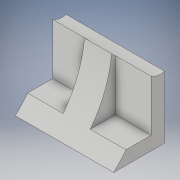
# Autodesk Inventor part: BottomRamp
Saved by Autodesk Inventor 2019 (Build 230136000, 136)
## iProperties
Created: 2020-01-13
Part Number: BottomRamp
Material: Generic
Document SubType Name: Modeling
Designer: james
Density: 1 g/cm^3
Appearance: Default
Author: james
Autodesk Inventor part; units mm, degrees
ref_plane "YZ Plane" through (0, 0, 0) normal (1, 0, 0) x (0, 1, 0)
ref_plane "XZ Plane" through (0, 0, 0) normal (0, 1, 0) x (-1, 0, 0)
ref_plane "XY Plane" through (0, 0, 0) normal (0, 0, 1) x (1, 0, 0)
sketch "Sketch1" plane through (0, 0, 0) normal (1, 0, 0) x (0, 1, 0)
  circle A0 centre (180.7797, 284.5338) radius 25.4
  line L0 (-17.3403, 309.9338) -> (-51.2615, 309.9338)
  line L1 (-51.2615, 309.9338) -> (-51.2615, -502.8662)
  line L2 (-51.2615, -502.8662) -> (-17.3403, -502.8662)
  line L3 (-17.3403, -502.8662) -> (-17.3403, 309.9338)
  line L4 (33.4597, 146.4304) -> (33.4597, 50.9549)
  arc A1 (202.8525, 71.0418) -> (198.1508, 77.005) centre (180.7797, 58.4738) ccw
  line L5 (198.1508, 7.6738) -> (231.5797, 7.6738)
  line L6 (231.5797, 7.6738) -> (231.5797, 309.9338)
  line L7 (231.5797, 309.9338) -> (33.4597, 309.9338)
  line L8 (33.4597, 146.4304) -> (33.4597, 50.9549)
  line L9 (198.1508, 76.3549) -> (198.1508, 50.9549)
  line L10 (33.4597, 50.9549) -> (33.4597, 76.3549)
  line L11 (33.4597, 50.9549) -> (58.8597, 50.9549)
  line L12 (33.4597, 119.3221) -> (33.4597, 50.9549)
  line L13 (149.9329, 50.9549) -> (33.4597, 50.9549)
  arc A2 (231.5797, 89.0982) -> (-17.3403, 245.4929) centre (180.7797, 284.5338) ccw
  arc A3 (33.4597, 146.4304) -> (161.2998, 83.5456) centre (180.7797, 284.5338) ccw
  arc A4 (161.2998, 83.5456) -> (149.9329, 50.9549) centre (180.7797, 58.4738) ccw
  arc A5 (198.1508, 70.6079) -> (202.8525, 71.0418) centre (180.7797, 284.5338) ccw
  arc A6 (231.5797, 76.0023) -> (-17.3403, 201.9838) centre (180.7797, 284.5338) ccw
  point P0 (0, 0)
  dimension "d1" = 50.8
  dimension "d2" = 812.8
  dimension "d5" = 25.4
  dimension "d6" = 198.12
  dimension "d10" = 50.8
  dimension "d11" = 50.8
  dimension "d12" = 226.06
  dimension "d15" = 25.4
  dimension "d16" = 50.8
  dimension "d17" = 302.26
  dimension "d18" = 50.8
  constraints: 28 end point, 12 point on circle, 8 point on line, 7 centre point, 5 parallel, 3 horizontal, 2 perpendicular, 1 coincident, 1 vertical
  measures "d1" diameter of A0
  measures "d2" distance of L2.end L0.start
  measures "d5" distance from line of L0 A0.centre
  measures "d6" distance from line of L3 A0.centre
  measures "d10" distance between parallel lines of L3 L4
  measures "d11" diameter of A1
  measures "d12" distance of A2.centre A1.centre
  measures "d15" distance from line of L7 A2.centre
  measures "d16" distance from line of L5 A1.centre
  measures "d17" distance between parallel lines of L7 L5
  measures "d18" distance from line of L6 A1.centre
extrude "Extrusion1" add sketch "Sketch1" along normal blind 50.8 contours A3 A4 L13 L11 L4
sketch "Sketch2" plane through (50.8, 0, 0) normal (1, 0, 0) x (0, 0, -1)
  line L0 (-146.4304, 33.4597) -> (-50.9549, 33.4597) projected
  line L1 (-50.9549, 33.4597) -> (-146.4304, 33.4597)
  line L2 (-123.5641, 58.8597) -> (-76.3549, 58.8597)
  line L3 (-50.9549, 58.8597) -> (-50.9549, 33.4597)
  line L4 (-50.9549, 33.4597) -> (-76.3549, 33.4597)
  line L5 (-76.3549, 58.8597) -> (-76.3549, 154.5437)
  line L6 (-50.9549, 149.9329) -> (-50.9549, 33.4597)
  arc A0 (-146.4304, 33.4597) -> (-83.5456, 161.2998) centre (-284.5338, 180.7797) ccw projected
  arc A1 (-83.5456, 161.2998) -> (-50.9549, 149.9329) centre (-58.4738, 180.7797) ccw projected
  line L7 (-50.9549, 33.4597) -> (-50.9549, 149.9329) projected
  arc A2 (-76.3549, 154.5437) -> (-50.9549, 149.9329) centre (-58.4738, 180.7797) ccw
  arc A3 (-146.4304, 33.4597) -> (-123.5641, 58.8597) centre (-284.5338, 180.7797) ccw
  point P0 (0, 0)
  dimension "d30" = 25.4
  dimension "d31" = 25.4
  constraints: 12 end point, 7 point on circle, 2 centre point, 2 coincident, 2 horizontal, 2 parallel, 1 perpendicular
  measures "d30" distance between parallel lines of L0 L2
  measures "d31" distance between parallel lines of L5 L6
extrude "Extrusion2" add sketch "Sketch2" along normal blind 66.675 contours A0 L2 L5 A1 L6 L3 L0
sketch "Sketch3" plane through (0, 0, 0) normal (-1, 0, 0) x (0, 0, 1)
  line L0 (76.3549, 58.8597) -> (76.3549, 154.5437) projected
  arc A0 (50.9549, 149.9329) -> (83.5456, 161.2998) centre (58.4738, 180.7797) ccw projected
  line L1 (50.9549, 33.4597) -> (50.9549, 149.9329) projected
  line L2 (146.4304, 33.4597) -> (50.9549, 33.4597) projected
  arc A1 (83.5456, 161.2998) -> (146.4304, 33.4597) centre (284.5338, 180.7797) ccw projected
  line L3 (123.5641, 58.8597) -> (76.3549, 58.8597) projected
  line L4 (76.3549, 154.5437) -> (76.3549, 58.8597) projected
  line L5 (76.3549, 154.5437) -> (76.3549, 58.8597)
  line L6 (76.3549, 58.8597) -> (123.5641, 58.8597)
  line L7 (50.9549, 149.9329) -> (50.9549, 33.4597)
  line L8 (146.4304, 33.4597) -> (50.9549, 33.4597)
  arc A2 (50.9549, 149.9329) -> (76.3549, 154.5437) centre (58.4738, 180.7797) ccw
  arc A3 (123.5641, 58.8597) -> (146.4304, 33.4597) centre (284.5338, 180.7797) ccw
  point P0 (0, 0)
  constraints: 8 end point, 4 point on circle, 2 centre point, 2 coincident, 2 collinear, 1 perpendicular, 1 vertical
extrude "Extrusion3" add sketch "Sketch3" along normal blind 66.675 contours L3 A1 L2 L1 A0 L0
body "Solid1"
